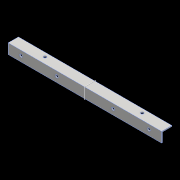
# Autodesk Inventor part: Lbarx1 small
Saved by Autodesk Inventor 2016 (Build 200138000, 138)
## iProperties
Created: 2019-02-12
Part Number: Lbarx1 small
Material: Aluminum 6061
Document SubType Name: Modeling
Designer: Calb3e
Density: 2.7 g/cm^3
Appearance: Aluminum - Flat
Author: Calb3e
Autodesk Inventor part; units mm, degrees
ref_plane "XZ Plane" through (0, 0, 0) normal (0, 1, 0) x (-1, 0, 0)
ref_plane "XY Plane" through (0, 0, 0) normal (0, 0, 1) x (1, 0, 0)
sketch "Sketch1" plane through (0, 0, 0) normal (0, 1, 0) x (-1, 0, 0)
  line L0 (0, 0) -> (-300, 0)
  line L1 (-300, 0) -> (-300, -20)
  line L2 (-300, -20) -> (0, -20)
  line L3 (0, -20) -> (0, 0)
  dimension "d0" = 300
  dimension "d1" = 20
  constraints: 8 end point, 2 parallel, 1 horizontal, 1 perpendicular
  measures "d0" distance of L0.start L0.end
  measures "d1" distance of L2.end L0.start
extrude "Extrusion1" add sketch "Sketch1" along normal blind 2
sketch "Sketch2" plane through (0, 2, 0) normal (0, 1, 0) x (1, 0, 0)
  line L0 (0, 0) -> (300, 0)
  line L1 (300, 0) -> (300, 2)
  line L2 (300, 2) -> (0, 2)
  line L3 (0, 2) -> (0, 0)
  dimension "d4" = 300
  dimension "d5" = 2
  constraints: 8 end point, 2 parallel, 1 horizontal, 1 perpendicular
  measures "d4" distance of L0.start L0.end
  measures "d5" distance of L2.end L0.start
extrude "Extrusion2" add sketch "Sketch2" along normal blind 18
hole "Hole1" at (60, 11.9755, 0) direction (0, 0, -1) diameter 5.5 end through all
pattern_linear "Rectangular Pattern1" count 2 spacing 190.136 along (1, 0, 0) of "Hole1"
hole "Hole2" at (25, 2, -9.3924) direction (0, -1, 0) diameter 5.5 end through all
pattern_linear "Rectangular Pattern2" count 2 spacing 70 along (1, 0, 0) of "Hole2"
ref_plane "Work Plane1" through (150, 0, 0) normal (1, 0, 0) x (0, 1, 0)
mirror "Mirror1" about plane through (150, 0, 0) normal (1, 0, 0) of "Hole2", "Rectangular Pattern2"
body "Solid1"
